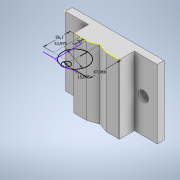
# Autodesk Inventor part: Soporte Superior Tubos
Saved by Autodesk Inventor 2021 (Build 250183000, 183)
## iProperties
Created: 2021-05-02
Part Number: Soporte Superior Tubos
Material: Generic
Document SubType Name: Modeling
Designer: maaro
Density: 1 g/cm^3
Appearance: Default
Author: maaro
Autodesk Inventor part; units mm, degrees
ref_plane "YZ Plane" through (0, 0, 0) normal (1, 0, 0) x (0, 1, 0)
ref_plane "XZ Plane" through (0, 0, 0) normal (0, 1, 0) x (-1, 0, 0)
ref_plane "XY Plane" through (0, 0, 0) normal (0, 0, 1) x (1, 0, 0)
sketch "Sketch2" plane through (0, 0, 0) normal (0, 0, 1) x (1, 0, 0)
  line L0 (0, 0) -> (200, 0)
  line L1 (200, 0) -> (200, 150)
  line L2 (200, 150) -> (0, 150)
  line L3 (0, 150) -> (0, 0)
  dimension "d4" = 150
  dimension "d5" = 200
  constraints: 8 end point, 2 parallel, 1 horizontal, 1 perpendicular
  measures "d4" distance of L2.end L0.start
  measures "d5" distance of L1.end L2.end
extrude "Extrusion2" add sketch "Sketch2" against normal blind 15
sketch "Sketch3" plane through (0, 0, 0) normal (0, 0, 1) x (1, 0, 0)
  line L0 (200, 150) -> (0, 150) projected
  line L1 (0, 150) -> (0, 0) projected
  point P0 (30, 75)
  point P1 (170, 75)
  dimension "d11" = 75
  dimension "d12" = 75
  dimension "d13" = 140
  dimension "d14" = 30
  measures "d11" distance from line of point (30, 75) L0
  measures "d12" distance from line of point (170, 75) L0
  measures "d13" distance of point (170, 75) point (30, 75)
  measures "d14" distance from line of point (30, 75) L1
hole "Hole1" at (30, 75, 0) at (170, 75, 0) direction (0, 0, -1) diameter 22.05 end through all
sketch "Sketch6" plane through (0, 150, 0) normal (0, 1, 0) x (1, 0, 0)
  line L0 (0, 0) -> (200, 0) projected
  line L1 (50, 0) -> (150, 0)
  line L2 (150, 0) -> (150, -32.5)
  line L3 (50, -32.5) -> (50, 0)
  line L4 (0, 0) -> (0, 15) projected
  line L5 (150, -32.5) -> (121.618, -32.5)
  line L6 (121.618, -32.5) -> (100, -25)
  line L7 (100, -25) -> (78.382, -32.5)
  line L8 (78.382, -32.5) -> (50, -32.5)
  dimension "d36" = 50
  dimension "d37" = 100
  dimension "d42" = 32.5
  dimension "d45" = 28.382
  dimension "d46" = 25
  constraints: 14 end point, 3 equal length, 3 point on line, 1 collinear, 1 horizontal, 1 vertical
  measures "d36" distance between parallel lines of L3 L4
  measures "d37" distance between parallel lines of L2 L3
  measures "d42" distance of L1.end L2.end
  measures "d45" distance of L2.end L5.end
  measures "d46" distance from line of L0 L6.end
extrude "Extrusion3" add sketch "Sketch6" against normal blind 150
chamfer "Chamfer1" distance 1 angle 45 2 edges at (150, 75, 32.5) (50, 75, 32.5)
sketch "Sketch7" plane through (0, 0, -15) normal (0, 0, -1) x (-1, 0, 0)
  line L0 (-100, 150) -> (-100, 0) projected
  line L1 (-200, 0) -> (0, 0) projected
  line L2 (0, 0) -> (0, 150) projected
  point P0 (-100, 75)
  dimension "d54" = 75
  dimension "d55" = 100
  constraints: 1 midpoint
  measures "d54" distance from line of L1 point (-100, 75)
  measures "d55" distance from line of L2 point (-100, 75)
hole "Hole3" at (100, 75, -15) direction (0, 0, 1) diameter 8.647 depth 25 tip angle 137 thread size "M10x1.25" class "6H" standard "ISO Metric profile"
sketch "Sketch8" plane through (0, 150, -15) normal (0, 1, 0) x (1, 0, 0)
  line L0 (78.382, -47.5) -> (78.382, -67.5) construction
  line L1 (78.382, -47.5) -> (51, -47.5) projected
  line L2 (100, -67.5) -> (100, -83.375)
  circle A0 centre (100, -94.4875) radius 26.9875
  line L3 (121.618, -47.5) -> (100, -40) projected
  line L4 (100, -67.5) -> (78.382, -67.5) construction
  line L5 (100, -121.475) -> (100, -94.4875) construction
  circle A1 centre (100, -113.5375) radius 7.9375
  line L6 (100, -105.6) -> (64.691, -105.6) construction
  line L7 (64.691, -105.6) -> (64.691, -47.5) construction
  line L8 (100, -40) -> (100, -121.475) construction
  line L9 (78.382, -47.5) -> (100, -40) projected
  line L10 (121.618, -47.5) -> (149, -47.5) projected
  line L11 (149, -115.4658) -> (121.8693, -115.4658)
  line L12 (121.8693, -115.4658) -> (100, -123.053)
  line L13 (100, -123.053) -> (78.1307, -115.4658)
  line L14 (78.1307, -115.4658) -> (51, -115.4658)
  line L15 (78.1307, -115.4658) -> (78.1307, -58.4908)
  point P0 (0, -15)
  dimension "d66" = 20
  dimension "d72" = 53.975
  dimension "d73" = 15.875
  dimension "d77" = 58.1
  dimension "d80" = 67.9658
  constraints: 24 end point, 4 point on circle, 4 point on line, 4 vertical, 2 centre point, 2 horizontal, 2 tangent, 1 collinear, 1 midpoint
  measures "d66" distance of L0.start L0.end
  measures "d72" diameter of A0
  measures "d73" diameter of A1
  measures "d77" distance of L6.end L7.end
  measures "d80" distance between parallel lines of L11 L10
equation "\"d12\" = d11"
body "Solid2"
